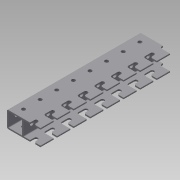
# Autodesk Inventor part: 9728
Saved by Autodesk Inventor 2013 (Build 170138000, 138)
## iProperties
Company: 80/20 Inc.
Created: 2014-04-23
Part Number: 9728
Material: Generic
Document SubType Name: Modeling
Density: 1 g/cm^3
Vendor: 80/20 Inc.
Engineer: Ross Bowman
Designer: Ross Bowman
Catalog Web Link: 8020.net
Material: 6105-T5 Aluminum
Author: Ross Bowman
Keywords: 80/20 , 8020 , T-Slot , Extrusion
Autodesk Inventor part; units mm, degrees
ref_plane "YZ Plane" through (0, 0, 0) normal (1, 0, 0) x (0, 1, 0)
ref_plane "XZ Plane" through (0, 0, 0) normal (0, 1, 0) x (-1, 0, 0)
ref_plane "XY Plane" through (0, 0, 0) normal (0, 0, 1) x (1, 0, 0)
sketch "Sketch1" plane through (0, 0, 0) normal (0, 0, 1) x (1, 0, 0)
  arc A0 (14.2748, -15.875) -> (15.875, -14.2748) centre (14.2748, -14.2748) ccw
  line L0 (15.875, -14.2748) -> (15.875, 14.2748)
  line L1 (14.2748, 15.875) -> (-14.2748, 15.875)
  arc A1 (-14.2748, 15.875) -> (-15.875, 14.2748) centre (-14.2748, 14.2748) ccw
  line L2 (-15.875, 14.2748) -> (-15.875, -14.2748)
  arc A2 (-15.875, -14.2748) -> (-14.2748, -15.875) centre (-14.2748, -14.2748) ccw
  line L3 (-14.2748, -15.875) -> (14.2748, -15.875)
  arc A3 (15.875, 14.2748) -> (14.2748, 15.875) centre (14.2748, 14.2748) ccw
  line L4 (-15.875, -19.05) -> (56.769, -19.05)
  line L5 (56.769, -19.05) -> (57.15, -18.669)
  line L6 (57.15, -18.669) -> (57.15, -16.256)
  line L7 (57.15, -16.256) -> (56.769, -15.875)
  line L8 (56.769, -15.875) -> (20.6502, -15.875)
  arc A4 (19.05, -14.2748) -> (20.6502, -15.875) centre (20.6502, -14.2748) ccw
  line L9 (19.05, -14.2748) -> (19.05, 14.2748)
  arc A5 (20.6502, 15.875) -> (19.05, 14.2748) centre (20.6502, 14.2748) ccw
  line L10 (20.6502, 15.875) -> (56.769, 15.875)
  line L11 (56.769, 15.875) -> (57.15, 16.256)
  line L12 (57.15, 16.256) -> (57.15, 18.669)
  line L13 (57.15, 18.669) -> (56.769, 19.05)
  line L14 (56.769, 19.05) -> (-15.875, 19.05)
  arc A6 (-15.875, 19.05) -> (-19.05, 15.875) centre (-15.875, 15.875) ccw
  line L15 (-19.05, 15.875) -> (-19.05, -15.875)
  arc A7 (-19.05, -15.875) -> (-15.875, -19.05) centre (-15.875, -15.875) ccw
  point P0 (0, 0)
  constraints: 32 end point, 16 point on circle, 8 centre point
extrude "Extrusion1" add sketch "Sketch1" against normal blind 304.8
hole "Hole1" at (-19.05, 0, -19.05) direction (1, 0, 0) diameter 8.3312 end through all
hole "Hole2" at (0, 19.05, -19.05) direction (0, -1, 0) diameter 8.3312 end through all
sketch "Sketch3" plane through (-15.875, 19.05, 0) normal (0, 1, 0) x (1, 0, 0)
  circle A0 centre (15.875, 19.05) radius 4.1656 projected
  line L0 (72.644, 0) -> (0, 0) projected
  line L1 (0, 0) -> (0, 304.8) projected
  line L2 (53.975, -7.3406) -> (73.025, -7.3406)
  line L3 (62.3062, 0.9906) -> (73.025, 0.9906)
  line L4 (73.025, 0.9906) -> (73.025, -7.3406)
  arc A1 (58.1406, 9.525) -> (49.8094, 9.5224) centre (53.975, 9.525) ccw
  circle A2 centre (49.8094, 9.525) radius 0.0026
  line L5 (49.8094, 9.525) -> (49.8094, -3.175)
  line L6 (58.1406, 9.525) -> (58.1406, 5.1562)
  arc A3 (58.1406, 5.1562) -> (62.3062, 0.9906) centre (62.3062, 5.1562) ccw
  arc A4 (49.8094, -3.175) -> (53.975, -7.3406) centre (53.975, -3.175) ccw
  line L7 (73.025, 0) -> (73.025, 304.8) projected
  point P0 (15.875, 0)
  dimension "d24" = 8.3312
  dimension "d25" = 4.1656
  dimension "d26" = 19.05
  dimension "d29" = 8.3312
  dimension "d33" = 38.1
  dimension "d37" = 12.7
  dimension "d38" = 8.3312
  dimension "d39" = 9.525
  constraints: 10 end point, 7 point on circle, 5 tangent, 3 centre point, 3 perpendicular, 2 parallel, 1 equal radius, 1 vertical alignment, 2 other
  measures "d24" diameter of A1
  measures "d25" radius of A3
  measures "d26" horizontal distance of L2.end A1.centre
  measures "d29" horizontal distance of A1.centre A3.centre
  measures "d33" horizontal distance of A1.centre A0.centre
  measures "d37" distance of A4.centre A1.centre
  measures "d38" distance of L3.end L2.end
  measures "d39" distance from line of L0 A1.centre
extrude "Extrusion2" cut sketch "Sketch3" against normal blind 50.8 contours A4 L5 A2 A1 L6 A3 L3 L4 L2 | A1 A2 picked at (49.811, 9.5246)
pattern_linear "Rectangular Pattern1" count 200 spacing 38.1 along (0, 0, -1) of "Hole2", "Hole1", "Extrusion2"
body "Solid1"
